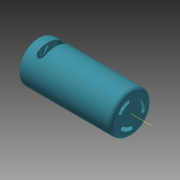
# Autodesk Inventor part: Motor housing
Saved by Autodesk Inventor 2015 (Build 190141000, 141)
## iProperties
Created: 2008-06-07
Part Number: Motor housing
Document SubType Name: Modeling
Designer: tangg
Density: 1.13 g/cm^3
Mass: 14.7217 g
Surface Area: 216.806 cm^2
Volume: 14.7217 cm^3
Stock Number: Motor housing
Material: Nylon-6/6
Appearance: Cadet Blue
Author: tangg
Autodesk Inventor part; units mm, degrees
ref_plane "YZ Plane" through (0, 0, 0) normal (1, 0, 0) x (0, 1, 0)
sketch "Sketch1" plane through (0, 0, 0) normal (0, 0, 1) x (1, 0, 0)
  line L0 (0, 0) -> (82.55, 0)
  line L1 (0, 0) -> (0, 18.5031)
  line L2 (82.55, 18.5031) -> (82.55, 0)
  line L3 (82.55, 18.5031) -> (82.55, 9.2516)
  line L4 (0, 18.5031) -> (82.55, 18.5031)
  point P0 (76.6061, 0)
  dimension "d13" = 82.55
  constraints: 10 end point, 2 horizontal, 2 vertical, 1 midpoint, 1 point on line
  measures "d13" distance of L1.end L2.start
revolve "Revolution1" add sketch "Sketch1" angle 360 about axis through (0, 0, 0) along (1, 0, 0)
fillet "Fillet1" radius 3.175 1 edges at (82.55, -18.5031, 0)
shell "Shell1" thickness 1.27 removed faces 1 at (0, 2.1153, -11.6887)
sketch "Sketch3" plane through (82.55, 0, 0) normal (1, 0, 0) x (0, 0, -1)
  arc A0 (9.2004, -2.4653) -> (8.2489, 4.7625) centre (0, 0) ccw
  arc A1 (12.2673, -3.287) -> (10.9985, 6.35) centre (0, 0) ccw
  line L0 (0, 0) -> (10.9985, 6.35) construction
  line L1 (0, 0) -> (12.2673, -3.287) construction
  line L2 (8.2489, 4.7625) -> (10.9985, 6.35)
  line L3 (9.2004, -2.4653) -> (12.2673, -3.287)
  circle A2 centre (9.6237, 5.5562) radius 1.5875
  circle A3 centre (10.7339, -2.8761) radius 1.5875
  dimension "d2" = 45
  constraints: 8 end point, 6 point on circle, 3 centre point, 2 coincident, 2 midpoint, 2 point on line, 3 other
  measures "d2" angle of L1 L0
extrude "Extrusion1" cut sketch "Sketch3" against normal blind 2.54
ref_plane "Work Plane2" through (78.74, 0, 0) normal (1, 0, 0) x (0, 0, -1)
sketch "Sketch4" plane through (78.74, 0, 0) normal (1, 0, 0) x (0, 0, -1)
  point P0 (0, 0)
pattern_circular "Circular Pattern1" count 3 over 360 about axis through (0, 0, 0) along (1, 0, 0) of "Extrusion1"
sketch "Sketch5" plane through (78.74, 0, 0) normal (1, 0, 0) x (0, 0, -1)
  point P0 (0, 0)
sketch "Sketch6" plane through (0, 0, 0) normal (-1, 0, 0) x (0, 0, 1)
  circle A0 centre (0, 0) radius 17.2331 projected
  circle A1 centre (0, 0) radius 18.5031 projected
extrude "Extrusion2" add sketch "Sketch6" along normal blind 2.54 contours A0 | A1
fillet "Fillet2" radius 3.175 1 edges at (-2.54, 0, -18.5031)
sketch "Sketch7" plane through (0, 0, 0) normal (0, 1, 0) x (-1, 0, 0)
  line L0 (-6.9464, 8.998) -> (-6.9464, -8.998)
  line L1 (16.51, 0) -> (-99.06, 0) projected
  line L2 (-13.6149, 8.7312) -> (-13.6149, -8.7312)
  arc A0 (-6.9464, 8.998) -> (-13.6149, 8.7312) centre (-10.2899, 9.0951) ccw
  arc A1 (-13.6149, -8.7312) -> (-6.9464, -8.998) centre (-10.2753, -8.7313) ccw
  point P0 (0, 0)
  point P1 (-6.9464, 0)
  point P2 (-13.6149, 0)
  constraints: 4 end point, 4 point on circle, 2 centre point, 2 midpoint, 2 point on line
extrude "Extrusion3" cut sketch "Sketch7" along normal through all both and the other way through all
ref_plane "Work Plane4" through (41.275, -9.2516, -16.0242) normal (0, -0.5, -0.8660254) x (1, 0, 0)
ref_plane "Work Plane3" through (0, 0, 0) normal (0, 0.5, 0.8660254) x (1, 0, 0)
sketch "Sketch8" plane through (41.275, -9.2516, -16.0242) normal (0, -0.5, -0.8660254) x (1, 0, 0)
  line L0 (26.9875, -22.225) -> (6.5654, -22.1959) construction
  line L1 (6.5654, -22.1959) -> (6.57, -19.0096) construction
  line L2 (6.57, -19.0096) -> (26.992, -19.0387) construction
  line L3 (26.992, -19.0387) -> (26.9875, -22.225) construction
  spline S0 degree 2 poles (24.2777, -20.6255) (24.2783, -20.2081) (24.6176, -19.5367) (24.902, -19.3494) knots 0 0 0 1 2 2 2
  spline S1 degree 2 poles (24.902, -19.3494) (25.1344, -19.204) (25.6112, -19.1059) (25.9817, -19.1064) knots 0 0 0 1 2 2 2
  line L4 (25.9817, -19.1064) -> (26.6832, -19.1074)
  line L5 (26.6832, -19.1074) -> (26.6788, -22.1554)
  line L6 (26.6788, -22.1554) -> (25.9848, -22.1544)
  spline S2 degree 2 poles (25.9848, -22.1544) (25.555, -22.1538) (25.0661, -22.0247) (24.8934, -21.9108) knots 0 0 0 1 2 2 2
  spline S3 degree 2 poles (24.8934, -21.9108) (24.5997, -21.7152) (24.2771, -21.0701) (24.2777, -20.6255) knots 0 0 0 1 2 2 2
  spline S4 degree 2 poles (24.7001, -20.631) (24.6996, -20.9818) (24.931, -21.4786) (25.1605, -21.6197) knots 0 0 0 1 2 2 2
  spline S5 degree 2 poles (25.1605, -21.6197) (25.3234, -21.7163) (25.6913, -21.8032) (25.9655, -21.8036) knots 0 0 0 1 2 2 2
  line L7 (25.9655, -21.8036) -> (26.2743, -21.8041)
  line L8 (26.2743, -21.8041) -> (26.2776, -19.4576)
  line L9 (26.2776, -19.4576) -> (25.9689, -19.4571)
  spline S6 degree 2 poles (25.9689, -19.4571) (25.6996, -19.4567) (25.292, -19.5426) (25.1263, -19.6585) knots 0 0 0 1 2 2 2
  spline S7 degree 2 poles (25.1263, -19.6585) (24.9137, -19.8014) (24.7006, -20.2754) (24.7001, -20.631) knots 0 0 0 1 2 2 2
  spline S8 degree 2 poles (22.9906, -19.0478) (23.3216, -19.0483) (23.7857, -19.1873) (23.9906, -19.2863) knots 0 0 0 1 2 2 2
  line L10 (23.9906, -19.2863) -> (23.9899, -19.7952)
  line L11 (23.9899, -19.7952) -> (23.9603, -19.7951)
  spline S9 degree 2 poles (23.9603, -19.7951) (23.7604, -19.6071) (23.2544, -19.3989) (23.0197, -19.3986) knots 0 0 0 1 2 2 2
  spline S10 degree 2 poles (23.0197, -19.3986) (22.6838, -19.3981) (22.3401, -19.6767) (22.3398, -19.9064) knots 0 0 0 1 2 2 2
  spline S11 degree 2 poles (22.3398, -19.9064) (22.3395, -20.0892) (22.5195, -20.3167) (22.7145, -20.3738) knots 0 0 0 1 2 2 2
  spline S12 degree 2 poles (22.7145, -20.3738) (22.8553, -20.4135) (23.0898, -20.4682) (23.2652, -20.5129) knots 0 0 0 1 2 2 2
  spline S13 degree 2 poles (23.2652, -20.5129) (23.4232, -20.5551) (23.6725, -20.6815) (23.7687, -20.7829) knots 0 0 0 1 2 2 2
  spline S14 degree 2 poles (23.7687, -20.7829) (23.8624, -20.8843) (23.9657, -21.1561) (23.9655, -21.334) knots 0 0 0 1 2 2 2
  spline S15 degree 2 poles (23.9655, -21.334) (23.9649, -21.7045) (23.3862, -22.205) (22.9392, -22.2044) knots 0 0 0 1 2 2 2
  spline S16 degree 2 poles (22.9392, -22.2044) (22.6823, -22.204) (22.2279, -22.1021) (22.033, -22.0055) knots 0 0 0 1 2 2 2
  line L12 (22.033, -22.0055) -> (22.0336, -21.5214)
  line L13 (22.0336, -21.5214) -> (22.0633, -21.5214)
  spline S17 degree 2 poles (22.0633, -21.5214) (22.2088, -21.655) (22.663, -21.8533) (22.9125, -21.8536) knots 0 0 0 1 2 2 2
  spline S18 degree 2 poles (22.9125, -21.8536) (23.1941, -21.854) (23.5427, -21.5902) (23.543, -21.3753) knots 0 0 0 1 2 2 2
  spline S19 degree 2 poles (23.543, -21.3753) (23.5433, -21.1827) (23.3386, -20.9527) (23.146, -20.9005) knots 0 0 0 1 2 2 2
  spline S20 degree 2 poles (23.146, -20.9005) (23.0176, -20.8658) (22.6448, -20.7763) (22.5214, -20.7391) knots 0 0 0 1 2 2 2
  spline S21 degree 2 poles (22.5214, -20.7391) (22.2078, -20.6423) (21.9169, -20.2541) (21.9173, -19.9701) knots 0 0 0 1 2 2 2
  spline S22 degree 2 poles (21.9173, -19.9701) (21.9176, -19.7897) (22.0638, -19.4441) (22.1949, -19.3233) knots 0 0 0 1 2 2 2
  spline S23 degree 2 poles (22.1949, -19.3233) (22.3408, -19.1901) (22.7115, -19.0474) (22.9906, -19.0478) knots 0 0 0 1 2 2 2
  spline S24 degree 2 poles (19.6934, -20.6214) (19.6945, -19.8014) (20.1723, -19.0339) (20.6688, -19.0346) knots 0 0 0 1 2 2 2
  spline S25 degree 2 poles (20.6688, -19.0346) (21.1727, -19.0353) (21.6433, -19.819) (21.6422, -20.6217) knots 0 0 0 1 2 2 2
  spline S26 degree 2 poles (21.6422, -20.6217) (21.641, -21.4467) (21.1632, -22.2093) (20.6643, -22.2086) knots 0 0 0 1 2 2 2
  spline S27 degree 2 poles (20.6643, -22.2086) (20.1629, -22.2079) (19.6922, -21.4168) (19.6934, -20.6214) knots 0 0 0 1 2 2 2
  spline S28 degree 2 poles (20.2183, -19.6935) (20.1588, -19.844) (20.1088, -20.3083) (20.1083, -20.622) knots 0 0 0 1 2 2 2
  spline S29 degree 2 poles (20.1083, -20.622) (20.1079, -20.9357) (20.1566, -21.3977) (20.2181, -21.5534) knots 0 0 0 1 2 2 2
  spline S30 degree 2 poles (20.2181, -21.5534) (20.2797, -21.7091) (20.4943, -21.8699) (20.6648, -21.8702) knots 0 0 0 1 2 2 2
  spline S31 degree 2 poles (20.6648, -21.8702) (20.8352, -21.8704) (21.0552, -21.7102) (21.1197, -21.5497) knots 0 0 0 1 2 2 2
  spline S32 degree 2 poles (21.1197, -21.5497) (21.1817, -21.3942) (21.2268, -20.92) (21.2272, -20.6212) knots 0 0 0 1 2 2 2
  spline S33 degree 2 poles (21.2272, -20.6212) (21.2277, -20.3001) (21.1888, -19.8702) (21.1248, -19.7022) knots 0 0 0 1 2 2 2
  spline S34 degree 2 poles (21.1248, -19.7022) (21.0657, -19.544) (20.8462, -19.3732) (20.6683, -19.373) knots 0 0 0 1 2 2 2
  spline S35 degree 2 poles (20.6683, -19.373) (20.5004, -19.3728) (20.2803, -19.533) (20.2183, -19.6935) knots 0 0 0 1 2 2 2
  spline S36 degree 2 poles (18.384, -19.0264) (18.6113, -19.0267) (18.9841, -19.1631) (19.1148, -19.2893) knots 0 0 0 1 2 2 2
  spline S37 degree 2 poles (19.1148, -19.2893) (19.2431, -19.413) (19.376, -19.7491) (19.3757, -19.9393) knots 0 0 0 1 2 2 2
  spline S38 degree 2 poles (19.3757, -19.9393) (19.3753, -20.1863) (19.1105, -20.6008) (18.8583, -20.724) knots 0 0 0 1 2 2 2
  line L14 (18.8583, -20.724) -> (18.8583, -20.7363)
  spline S39 degree 2 poles (18.8583, -20.7363) (19.0829, -20.8676) (19.2998, -21.1791) (19.2995, -21.4113) knots 0 0 0 1 2 2 2
  spline S40 degree 2 poles (19.2995, -21.4113) (19.299, -21.7546) (18.7796, -22.2133) (18.3795, -22.2127) knots 0 0 0 1 2 2 2
  spline S41 degree 2 poles (18.3795, -22.2127) (17.9645, -22.2121) (17.4637, -21.7767) (17.4642, -21.4358) knots 0 0 0 1 2 2 2
  spline S42 degree 2 poles (17.4642, -21.4358) (17.4645, -21.2308) (17.7047, -20.831) (17.9296, -20.7177) knots 0 0 0 1 2 2 2
  line L15 (17.9296, -20.7177) -> (17.9296, -20.7054)
  spline S43 degree 2 poles (17.9296, -20.7054) (17.6631, -20.5815) (17.3894, -20.2254) (17.3898, -19.9438) knots 0 0 0 1 2 2 2
  spline S44 degree 2 poles (17.3898, -19.9438) (17.3903, -19.5536) (17.9592, -19.0258) (18.384, -19.0264) knots 0 0 0 1 2 2 2
  spline S45 degree 2 poles (17.8097, -19.9049) (17.8095, -20.0926) (17.9574, -20.3151) (18.1672, -20.4291) knots 0 0 0 1 2 2 2
  spline S46 degree 2 poles (18.1672, -20.4291) (18.2363, -20.4687) (18.4683, -20.5604) (18.614, -20.6199) knots 0 0 0 1 2 2 2
  spline S47 degree 2 poles (18.614, -20.6199) (18.7821, -20.509) (18.9629, -20.1783) (18.9632, -19.9683) knots 0 0 0 1 2 2 2
  spline S48 degree 2 poles (18.9632, -19.9683) (18.9636, -19.6917) (18.6306, -19.3306) (18.3787, -19.3302) knots 0 0 0 1 2 2 2
  spline S49 degree 2 poles (18.3787, -19.3302) (18.1218, -19.3298) (17.8101, -19.6382) (17.8097, -19.9049) knots 0 0 0 1 2 2 2
  spline S50 degree 2 poles (17.8644, -21.4315) (17.8641, -21.6365) (18.1379, -21.911) (18.3824, -21.9114) knots 0 0 0 1 2 2 2
  spline S51 degree 2 poles (18.3824, -21.9114) (18.6047, -21.9117) (18.8891, -21.6676) (18.8894, -21.4576) knots 0 0 0 1 2 2 2
  spline S52 degree 2 poles (18.8894, -21.4576) (18.8896, -21.307) (18.7442, -21.0968) (18.5986, -21.0126) knots 0 0 0 1 2 2 2
  spline S53 degree 2 poles (18.5986, -21.0126) (18.5369, -20.9779) (18.2752, -20.8565) (18.1691, -20.8218) knots 0 0 0 1 2 2 2
  spline S54 degree 2 poles (18.1691, -20.8218) (17.991, -20.9574) (17.8646, -21.2462) (17.8644, -21.4315) knots 0 0 0 1 2 2 2
  spline S55 degree 2 poles (15.09, -20.0789) (15.0903, -19.8442) (15.2465, -19.4468) (15.3776, -19.3136) knots 0 0 0 1 2 2 2
  spline S56 degree 2 poles (15.3776, -19.3136) (15.5137, -19.173) (15.8547, -19.0277) (16.0598, -19.028) knots 0 0 0 1 2 2 2
  spline S57 degree 2 poles (16.0598, -19.028) (16.2648, -19.0283) (16.603, -19.1671) (16.7312, -19.3056) knots 0 0 0 1 2 2 2
  spline S58 degree 2 poles (16.7312, -19.3056) (16.8891, -19.4713) (17.0661, -20.0274) (17.0655, -20.4324) knots 0 0 0 1 2 2 2
  spline S59 degree 2 poles (17.0655, -20.4324) (17.065, -20.8301) (16.901, -21.4696) (16.7303, -21.7065) knots 0 0 0 1 2 2 2
  spline S60 degree 2 poles (16.7303, -21.7065) (16.5644, -21.9384) (16.0404, -22.197) (15.6971, -22.1965) knots 0 0 0 1 2 2 2
  spline S61 degree 2 poles (15.6971, -22.1965) (15.5958, -22.1964) (15.418, -22.1764) (15.3513, -22.1541) knots 0 0 0 1 2 2 2
  line L16 (15.3513, -22.1541) -> (15.3519, -21.7613)
  line L17 (15.3519, -21.7613) -> (15.3692, -21.7614)
  spline S62 degree 2 poles (15.3692, -21.7614) (15.426, -21.7911) (15.6334, -21.8432) (15.7519, -21.8434) knots 0 0 0 1 2 2 2
  spline S63 degree 2 poles (15.7519, -21.8434) (16.1323, -21.844) (16.5999, -21.3309) (16.6451, -20.827) knots 0 0 0 1 2 2 2
  spline S64 degree 2 poles (16.6451, -20.827) (16.4992, -20.9281) (16.1927, -21.0388) (16.01, -21.0386) knots 0 0 0 1 2 2 2
  spline S65 degree 2 poles (16.01, -21.0386) (15.8321, -21.0383) (15.5655, -20.9663) (15.4199, -20.8574) knots 0 0 0 1 2 2 2
  spline S66 degree 2 poles (15.4199, -20.8574) (15.2521, -20.7312) (15.0896, -20.3407) (15.09, -20.0789) knots 0 0 0 1 2 2 2
  spline S67 degree 2 poles (15.505, -20.0622) (15.5047, -20.2499) (15.6032, -20.5045) (15.7117, -20.5935) knots 0 0 0 1 2 2 2
  spline S68 degree 2 poles (15.7117, -20.5935) (15.7931, -20.6579) (15.9956, -20.7001) (16.1018, -20.7003) knots 0 0 0 1 2 2 2
  spline S69 degree 2 poles (16.1018, -20.7003) (16.2451, -20.7005) (16.5144, -20.6144) (16.6455, -20.5331) knots 0 0 0 1 2 2 2
  spline S70 degree 2 poles (16.6455, -20.5331) (16.648, -20.4887) (16.6531, -20.4047) (16.6532, -20.3405) knots 0 0 0 1 2 2 2
  spline S71 degree 2 poles (16.6532, -20.3405) (16.6536, -20.0243) (16.5307, -19.6363) (16.4369, -19.5349) knots 0 0 0 1 2 2 2
  spline S72 degree 2 poles (16.4369, -19.5349) (16.3506, -19.4385) (16.163, -19.3616) (16.0568, -19.3615) knots 0 0 0 1 2 2 2
  spline S73 degree 2 poles (16.0568, -19.3615) (15.8098, -19.3611) (15.5055, -19.7114) (15.505, -20.0622) knots 0 0 0 1 2 2 2
  line L18 (13.0043, -19.0879) -> (14.4912, -19.09)
  line L19 (14.4912, -19.09) -> (14.4908, -19.4012)
  line L20 (14.4908, -19.4012) -> (13.9375, -19.4004)
  line L21 (13.9375, -19.4004) -> (13.9346, -21.4431)
  line L22 (13.9346, -21.4431) -> (14.4878, -21.4439)
  line L23 (14.4878, -21.4439) -> (14.4875, -21.723)
  spline S74 degree 2 poles (14.4875, -21.723) (14.1738, -21.7226) (13.8771, -21.9) (13.857, -22.147) knots 0 0 0 1 2 2 2
  line L24 (13.857, -22.147) -> (13.5408, -22.1465)
  line L25 (13.5408, -22.1465) -> (13.5447, -19.3999)
  line L26 (13.5447, -19.3999) -> (13.0038, -19.3991)
  line L27 (13.0038, -19.3991) -> (13.0043, -19.0879)
  line L28 (11.3255, -20.2341) -> (12.479, -20.2357)
  line L29 (12.479, -20.2357) -> (12.4784, -20.6062)
  line L30 (12.4784, -20.6062) -> (11.325, -20.6046)
  line L31 (11.325, -20.6046) -> (11.3255, -20.2341)
  line L32 (8.9594, -20.1294) -> (9.3224, -20.1299)
  line L33 (9.3224, -20.1299) -> (9.3239, -19.0826)
  line L34 (9.3239, -19.0826) -> (9.7167, -19.0832)
  line L35 (9.7167, -19.0832) -> (9.7152, -20.1305)
  line L36 (9.7152, -20.1305) -> (11.0613, -20.1324)
  line L37 (11.0613, -20.1324) -> (11.0607, -20.5622)
  line L38 (11.0607, -20.5622) -> (9.695, -22.1312)
  line L39 (9.695, -22.1312) -> (9.3196, -22.1306)
  line L40 (9.3196, -22.1306) -> (9.322, -20.4584)
  line L41 (9.322, -20.4584) -> (8.9589, -20.4579)
  line L42 (8.9589, -20.4579) -> (8.9594, -20.1294)
  line L43 (9.7147, -20.459) -> (9.713, -21.6495)
  line L44 (9.713, -21.6495) -> (10.7398, -20.4605)
  line L45 (10.7398, -20.4605) -> (9.7147, -20.459)
  line L46 (6.6721, -20.1261) -> (7.0352, -20.1267)
  line L47 (7.0352, -20.1267) -> (7.0367, -19.0794)
  line L48 (7.0367, -19.0794) -> (7.4294, -19.0799)
  line L49 (7.4294, -19.0799) -> (7.4279, -20.1272)
  line L50 (7.4279, -20.1272) -> (8.7741, -20.1291)
  line L51 (8.7741, -20.1291) -> (8.7735, -20.5589)
  line L52 (8.7735, -20.5589) -> (7.4078, -22.1279)
  line L53 (7.4078, -22.1279) -> (7.0324, -22.1274)
  line L54 (7.0324, -22.1274) -> (7.0347, -20.4552)
  line L55 (7.0347, -20.4552) -> (6.6717, -20.4547)
  line L56 (6.6717, -20.4547) -> (6.6721, -20.1261)
  line L57 (7.4275, -20.4557) -> (7.4258, -21.6463)
  line L58 (7.4258, -21.6463) -> (8.4525, -20.4572)
  line L59 (8.4525, -20.4572) -> (7.4275, -20.4557)
  point P0 (-41.275, 0)
  dimension "d17" = 3.1863
  dimension "d18" = 20.4221
  constraints: 2 other
  measures "d17" distance of L0.end L1.end
  measures "d18" distance of L1.end L2.end
emboss "Emboss1" sketch "Sketch8" operation cut depth 0.254 direction (0, 0.5, 0.8660254) wrap yes faces at (30.2719, -11.7847, -14.2649)
sketch "Sketch9" plane through (-2.54, 0, 0) normal (-1, 0, 0) x (0, 0, 1)
  line L0 (0, 0) -> (1.1674, 14.8333) construction
  line L1 (0, 0) -> (-1.266, 16.0858) construction
  line L2 (0, 25.9044) -> (0, -25.9044) construction
  circle A0 centre (0, 0) radius 4.7625 construction
  circle A1 centre (0, 0) radius 11.1469 construction
  line L3 (-0.3737, 4.7478) -> (-0.8746, 11.1125)
  line L4 (0.3737, 4.7478) -> (0.8746, 11.1125)
  arc A2 (0.8746, 11.1125) -> (-0.8746, 11.1125) centre (0, 0) ccw
  arc A3 (0.3737, 4.7478) -> (-0.3737, 4.7478) centre (0, 0) ccw
  dimension "d21" = 9
  dimension "d22" = 4.5
  constraints: 8 end point, 6 point on circle, 4 point on line, 3 centre point, 2 coincident, 3 other
  measures "d21" angle of L0 L1
  measures "d22" angle of L0 L2
extrude "Extrusion4" cut sketch "Sketch9" against normal up to next
pattern_circular "Circular Pattern2" count 10 over 360 about axis through (41.275, 0, 0) along (1, 0, 0) of "Extrusion4"
body "Solid1"
